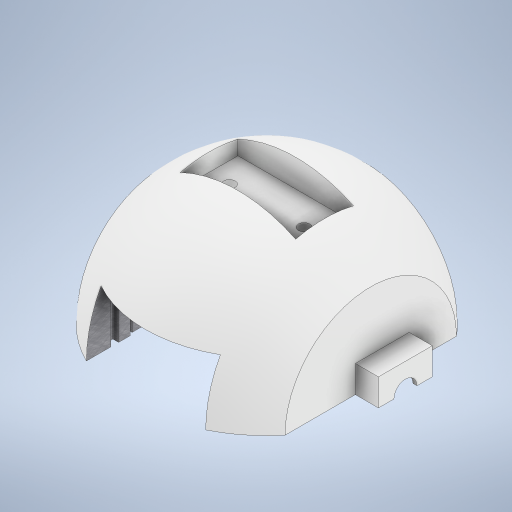
# Autodesk Inventor part: naibu-rightside
Saved by Autodesk Inventor 2023 (Build 270158000, 158)
## iProperties
Created: 2022-10-08
Part Number: naibu-rightside
Material: ABS プラスチック
Document SubType Name: Modeling
Designer: ellie
Density: 1.06 g/cm^3
Appearance: 積雪
Author: ellie
Autodesk Inventor part; units mm, degrees
ref_plane "YZ Plane" through (0, 0, 0) normal (1, 0, 0) x (0, 1, 0)
ref_plane "XZ Plane" through (0, 0, 0) normal (0, 1, 0) x (-1, 0, 0)
ref_plane "XY Plane" through (0, 0, 0) normal (0, 0, 1) x (1, 0, 0)
sketch "スケッチ1" plane through (0, 0, 0) normal (0, 1, 0) x (-1, 0, 0)
  circle A0 centre (0, 0) radius 35
  line L0 (0, 0) -> (0, -35)
  line L1 (0, 0) -> (0, 35)
  dimension "d0" = 70
  constraints: 4 end point, 2 point on circle, 2 vertical, 1 centre point, 1 coincident
  measures "d0" diameter of A0
revolve "回転1" add sketch "スケッチ1" angle 180 about axis through (0, 0, 0) along (0, 0, 1) picked at (-2.5961, -23.0408) contours L1 L0 A0
sketch "スケッチ5" plane through (0, 0, 0) normal (0, -1, 0) x (1, 0, 0)
  line L0 (-20, -23) -> (20, -23)
  line L1 (20, -23) -> (20, -13)
  line L2 (20, -13) -> (-20, -13)
  line L3 (-20, -13) -> (-20, -23)
  line L4 (-20, -15) -> (-20, -13)
  line L5 (0, 25) -> (-17, 25)
  line L6 (-17, 25) -> (-17, 23)
  line L7 (-17, 23) -> (0, 23)
  line L8 (0, 23) -> (0, 25)
  line L9 (0, 20) -> (-20, 20)
  line L10 (-20, 20) -> (-20, 19)
  line L11 (-20, 19) -> (0, 19)
  line L12 (0, 19) -> (0, 20)
  line L13 (0, 13) -> (-19, 13)
  line L14 (-19, 13) -> (-19, 11)
  line L15 (-19, 11) -> (0, 11)
  line L16 (0, 11) -> (0, 13)
  line L17 (0, 5) -> (-23, 5)
  line L18 (-23, 5) -> (-23, 3)
  line L19 (-23, 3) -> (0, 3)
  line L20 (0, 3) -> (0, 5)
  circle A0 centre (0, 0) radius 35 projected
  circle A1 centre (0, 0) radius 35 projected
  line L21 (0, 35) -> (0, -35)
  line L22 (35, 0) -> (-35, 0)
  line L23 (-32, 2) -> (-23, 2)
  line L24 (-23, 2) -> (-23, -8)
  line L25 (-23, -8) -> (-32, -8)
  line L26 (-32, -8) -> (-32, 2)
  line L27 (-23, -8.0262) -> (-23, 2)
  line L28 (-27, 22.2711) -> (-27, -22.2711)
  line L29 (-15.5, 25) -> (0, 25)
  line L30 (0, 25) -> (0, 35)
  line L31 (0, 35) -> (-15.5, 35)
  line L32 (-15.5, 35) -> (-15.5, 25)
  line L33 (-15.5, 23) -> (0, 23)
  line L34 (0, 23) -> (0, 20)
  line L35 (0, 20) -> (-15.5, 20)
  line L36 (-15.5, 20) -> (-15.5, 23)
  line L37 (-16, 13) -> (0, 13)
  line L38 (0, 13) -> (0, 19)
  line L39 (0, 19) -> (-16, 19)
  line L40 (-16, 19) -> (-16, 13)
  line L41 (-16, 11) -> (0, 11)
  line L42 (0, 11) -> (0, 5)
  line L43 (0, 5) -> (-16, 5)
  line L44 (-16, 5) -> (-16, 11)
  line L45 (-23, -3) -> (-39.6865, -3)
  line L46 (-23, -3) -> (-7.8337, -3)
  line L47 (-8, 3) -> (-23, 3)
  line L48 (-23, 3) -> (-23, -9)
  line L49 (-23, -9) -> (-8, -9)
  line L50 (-8, -9) -> (-8, 3)
  line L51 (-8, 3) -> (-23, -9) construction
  line L52 (-23, 3) -> (-8, -9) construction
  line L53 (-23, 4) -> (-33, 4)
  line L54 (-33, 4) -> (-33, -10)
  line L55 (-33, -10) -> (-23, -10)
  line L56 (-23, -10) -> (-23, 4)
  line L57 (-23, 4) -> (-33, -10) construction
  line L58 (-33, 4) -> (-23, -10) construction
  line L59 (-8, 3) -> (-1, 3)
  line L60 (-1, 3) -> (-1, -9)
  line L61 (-1, -9) -> (-8, -9)
  line L62 (-8, -9) -> (-8, 3)
  line L63 (-8, 3) -> (-1, -9) construction
  line L64 (-1, 3) -> (-8, -9) construction
  line L65 (-23, 2) -> (-27, 2)
  line L66 (-23, -8) -> (-27, -8)
  line L67 (-23, 4) -> (-27, 4)
  line L68 (-23, -10) -> (-27, -10)
  line L69 (23.4307, -26) -> (-23.4307, -26)
  line L70 (-8, 3) -> (-6.8, 3)
  line L71 (-6.8, 3) -> (-6.8, -9)
  line L72 (-6.8, -9) -> (-8, -9)
  line L73 (-8, -9) -> (-8, 3)
  line L74 (0, 5) -> (2, 5)
  line L75 (0, -3) -> (0, 5)
  line L76 (-11.5791, -13) -> (-8, -13)
  point P0 (0, -23)
  point P1 (0, -13)
  point P2 (0, 24)
  point P3 (0, 19.5)
  point P4 (0, 12)
  point P5 (0, 4)
  point P6 (-20, -18)
  point P7 (-27, -0.5262)
  point P8 (-27, -8)
  point P9 (-15.5, 21.5)
  point P10 (-15.5, 31.3807)
  point P11 (0, 25)
  point P12 (0, 23)
  point P13 (0, 11)
  point P14 (0, 13)
  point P15 (-27, 0)
  point P16 (-32, 0)
  point P17 (-23, 0)
  point P18 (-15.5, -3)
  point P19 (-28, -3)
  point P20 (-4.5, -3)
  point P21 (-8, 3)
  point P22 (-27, 0.5)
  point P23 (-28, 0.4738)
  point P24 (-28, -11.5262)
  point P25 (-27, -11.5)
  point P26 (-23, 3)
  point P27 (-8, 0)
  point P28 (-1, 0)
  point P29 (-6.8, 3)
  point P30 (0, 5)
  point P31 (0, 3)
  point P32 (-27, -10)
  point P33 (-27, 4)
  dimension "d12" = 40
  dimension "d13" = 10
  dimension "d23" = 17
  dimension "d24" = 2
  dimension "d27" = 20
  dimension "d28" = 1
  dimension "d30" = 19
  dimension "d31" = 2
  dimension "d33" = 2
  dimension "d88" = 0
  dimension "d89" = 0
  dimension "d90" = 12
  dimension "d92" = 20
  dimension "d93" = 10
  dimension "d97" = 9
  dimension "d98" = 10
  dimension "d113" = 27
  dimension "d122" = 15.5
  dimension "d123" = 35
  dimension "d124" = 3
  dimension "d125" = 15.5
  dimension "d126" = 6
  dimension "d127" = 6
  dimension "d128" = 16
  dimension "d129" = 16
  dimension "d147" = 12
  dimension "d149" = 8
  dimension "d151" = 15
  dimension "d161" = 14
  dimension "d162" = 10
  dimension "d164" = 12
  dimension "d165" = 7
  dimension "d170" = 26
  dimension "d175" = 1.2
  dimension "d187" = 1
  constraints: 152 end point, 29 parallel, 19 horizontal, 17 perpendicular, 15 midpoint, 15 point on line, 9 collinear, 1 vertical, 20 other
  measures "d12" distance of L2.end L1.end
  measures "d13" distance of L1.end L0.end
  measures "d23" distance of L7.end L6.end
  measures "d24" distance of L6.end L5.end
  measures "d27" distance of L11.end L10.end
  measures "d28" distance of L10.end L9.end
  measures "d30" distance of L15.end L14.end
  measures "d31" distance of L14.end L13.end
  measures "d33" distance of L18.end L17.end
  measures "d89" distance from line of point (0, 0) L22
  measures "d90" distance from line of L0 point (0, -35)
  measures "d92" distance of the line from the sketch origin of L3
  measures "d93" distance from line of L5 point (0, 35)
  measures "d97" distance of L24.end L25.end
  measures "d98" distance of L23.end L24.end
  measures "d113" distance of the line from the sketch origin of L28
  measures "d122" distance of the line from the sketch origin of L32
  measures "d123" distance between parallel lines of L31 L22
  measures "d124" distance of L33.end L34.end
  measures "d126" distance of L38.end L37.end
  measures "d127" distance of L41.end L42.end
  measures "d128" distance of the line from the sketch origin of L44
  measures "d129" distance of the line from the sketch origin of L40
  measures "d147" distance of L48.end L47.end
  measures "d149" distance of the line from the sketch origin of L50
  measures "d151" distance between parallel lines of L50 L24
  measures "d161" distance between parallel lines of L55 L53
  measures "d162" distance between parallel lines of L48 L54
  measures "d164" distance between parallel lines of L61 L59
  measures "d165" distance between parallel lines of L50 L60
  measures "d170" distance between parallel lines of L69 L22
  measures "d175" distance of L71.end L72.end
  measures "d187" distance between parallel lines of L75 L60
extrude "GNSボード" cut sketch "スケッチ5" against normal blind 16 contours L8 L7 L6 L5
extrude "GNSボード止めるよう" cut sketch "スケッチ5" against normal blind 15 contours L21 L5 L32 A0 | L21 L9 L36 L7
extrude "アルミ板１" cut sketch "スケッチ5" against normal blind 20 contours L12 L11 L10 L9
extrude "メイン基板" cut sketch "スケッチ5" against normal blind 17.5 contours L15 L14 L13 L16
extrude "メイン止めるよう" cut sketch "スケッチ5" against normal blind 16.5 contours L17 L44 L15 L21 | L13 L40 L11 L21
extrude "アルミ板２" cut sketch "スケッチ5" against normal blind 17.5 contours L19 L18 L17 L20
extrude "電池ボックス入れ" cut sketch "スケッチ5" against normal blind 13 contours L3 L2 L21 L0 | L21 L2 L1 L0
extrude "side ut" cut sketch "スケッチ5" against normal blind 100 contours A0 L45 L54 L55 L28 | A0 L22 L54 L45 | L55 L54 L45 L26 L25 L28 | A0 L28 L53 L54 L22 | L54 L22 L26 L45 | L25 L26 L45 L28 | L54 L53 L28 L23 L26 L22 | L26 L22 L28 L45 | L26 L23 L28 L22
extrude "motor case" add sketch "スケッチ5" against normal blind 7 contours L55 L54 L45 L26 L25 L28 | L28 L25 L27 L48 L56 L55 | L54 L22 L26 L45 | L28 L45 L24 L25 | L25 L26 L45 L28 | L50 L46 L24 L22 | L22 L24 L48 L19 L50 | L54 L53 L28 L23 L26 L22 | L26 L22 L28 L45 | L24 L46 L50 L49 L48 L27 | L28 L22 L24 L45 | L22 L28 L23 L24 | L53 L18 L48 L23 L28 | L26 L23 L28 L22
extrude "bottom cut" cut sketch "スケッチ5" against normal blind 90 contours L69 A0 L21 | L21 A0 L69
extrude "motor" cut sketch "スケッチ5" against normal blind 6 contours L60 L61 L71 L22 | L22 L71 L19 L60 | L71 L61 L50 L22 | L22 L50 L19 L71 | L28 L45 L24 L25 | L25 L26 L45 L28 | L50 L46 L24 L22 | L22 L24 L48 L19 L50 | L26 L22 L28 L45 | L24 L46 L50 L49 L48 L27 | L28 L22 L24 L45 | L22 L28 L23 L24 | L26 L23 L28 L22
extrude "motor block" add sketch "スケッチ5" against normal blind 10 contours L71 L61 L50 L22 | L22 L50 L19 L71
sketch "スケッチ26" plane through (-33, 0, -10) normal (-1, 0, 0) x (0, 0, 1)
  line L0 (14, 0) -> (0, 0) projected
  circle A0 centre (7, 0) radius 3
  point P0 (10, 0)
  point P1 (7, 0)
  point P2 (4, 0)
  point P3 (10, 0)
  dimension "d197" = 6
  constraints: 1 centre point, 1 coincident
  measures "d197" diameter of A0
extrude "押し出し34" cut sketch "スケッチ26" against normal blind 27 contours L0 A0 picked at (7.7485, 0.6631)
mirror "ミラー11" about plane through (0, 0, 0) normal (1, 0, 0) of "GNSボード", "GNSボード止めるよう", "アルミ板１", "メイン止めるよう", "メイン基板", "アルミ板２", "motor", "押し出し34", "motor case", "電池ボックス入れ", "motor block", "side ut"
ref_plane "作業平面5" through (0, 13, 0) normal (0, -1, 0) x (1, 0, 0)
ref_plane "作業平面6" through (-15.5, 35, 25) normal (0, -1, 0) x (1, 0, 0)
sketch "スケッチ29" plane through (-15.5, 35, 25) normal (0, -1, 0) x (1, 0, 0)
  line L0 (15.5, -25) -> (-67.7134, -25)
  line L1 (-67.7134, -25) -> (15.5, -25)
  line L2 (110.7852, -24.5555) -> (110.7852, -27.3413)
  line L3 (15.5, -25) -> (98.1975, -25)
  circle A0 centre (25.2, -25) radius 1.5
  circle A1 centre (5.8, -25) radius 1.5
  line L4 (32.5, 0) -> (-1.5, 0) projected
  line L5 (15.5, 0) -> (15.5, -51)
  line L6 (-7.9307, -51) -> (38.9307, -51) projected
  dimension "d205" = 3
  dimension "d206" = 19.4
  dimension "d207" = 0
  constraints: 10 end point, 2 centre point, 2 horizontal, 2 midpoint, 1 collinear, 1 vertical, 1 other
  measures "d205" diameter of A0
  measures "d206" distance of A1.centre A0.centre
  measures "d207" distance from line of L3 A0.centre
extrude "押し出し36" cut sketch "スケッチ29" along normal up to surface (29 mm away)
sketch "スケッチ30" plane through (-15.5, 35, 25) normal (0, -1, 0) x (1, 0, 0)
  line L0 (0.5, -17.5) -> (30.5, -17.5)
  line L1 (30.5, -17.5) -> (30.5, -32.5)
  line L2 (30.5, -32.5) -> (0.5, -32.5)
  line L3 (0.5, -32.5) -> (0.5, -17.5)
  line L4 (0.5, -17.5) -> (30.5, -32.5) construction
  line L5 (30.5, -17.5) -> (0.5, -32.5) construction
  point P0 (15.5, -25)
  dimension "d210" = 30
  dimension "d211" = 15
  constraints: 12 end point, 2 midpoint, 2 parallel, 1 horizontal, 1 perpendicular
  measures "d210" distance of L1.end L2.end
  measures "d211" distance of L0.end L1.end
extrude "押し出し37" cut sketch "スケッチ30" along normal blind 8
